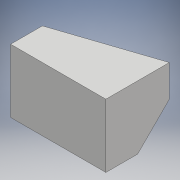
# Autodesk Inventor part: 14
Saved by Autodesk Inventor 2017 (Build 210142000, 142)
## iProperties
Part Number: 14
Material: 一般
Document SubType Name: Modeling
Designer: Brian
Density: 1 g/cm^3
Appearance: 預設
Author: Brian
Autodesk Inventor part; units mm, degrees
ref_plane "YZ Plane" through (0, 0, 0) normal (1, 0, 0) x (0, 1, 0)
ref_plane "XZ Plane" through (0, 0, 0) normal (0, 1, 0) x (-1, 0, 0)
sketch "草圖1" plane through (0, 0, 0) normal (0, 1, 0) x (-1, 0, 0)
  line L0 (0, 0) -> (-60, 0)
  line L1 (-60, 0) -> (-60, -40)
  line L2 (-60, -40) -> (0, -40)
  line L3 (0, -40) -> (0, 0)
  dimension "d0" = 40
  dimension "d1" = 60
  constraints: 8 end point, 2 parallel, 1 horizontal, 1 perpendicular
  measures "d0" distance of L2.end L0.start
  measures "d1" distance of L1.end L2.end
extrude "擠出1" add sketch "草圖1" along normal blind 40
sketch "草圖2" plane through (0, 0, -40) normal (-1, 0, 0) x (0, 0, 1)
  line L0 (40, 40) -> (0, 40) projected
  line L1 (20, 40) -> (40, 20)
  line L2 (40, 0) -> (40, 40) projected
  dimension "d4" = 20
  dimension "d5" = 20
  constraints: 2 end point, 2 midpoint
  measures "d4" distance of L0.start L1.start
  measures "d5" distance of L0.start L1.end
ref_plane "工作平面1" through (0, 40, -20) normal (-0.2294, 0.6882, 0.6882) x (0, -0.7071, 0.7071)
sketch "草圖3" plane through (0, 40, -20) normal (-0.2294, 0.6882, 0.6882) x (0, -0.7071, 0.7071)
  line L0 (-6.4039, -15.4846) -> (38.9012, -15.4846)
  line L1 (38.9012, -15.4846) -> (38.9012, 77.4757)
  line L2 (38.9012, 77.4757) -> (-6.4039, 77.4757)
  line L3 (-6.4039, 77.4757) -> (-6.4039, -15.4846)
  point P0 (42.4264, -3.2444)
  constraints: 8 end point, 2 parallel, 1 horizontal, 1 perpendicular
extrude "擠出2" cut sketch "草圖3" along normal blind 40
ref_plane "工作平面2" through (60, 0, -20) normal (0, 0, -1) x (-1, 0, 0)
ref_plane "工作平面3" through (30, 0, 0) normal (1, 0, 0) x (0, 0, -1)
pattern_circular "環形陣列1" count 2 over 360 about axis through (30, 0, -20) along (0, -1, 0) of "擠出2"
